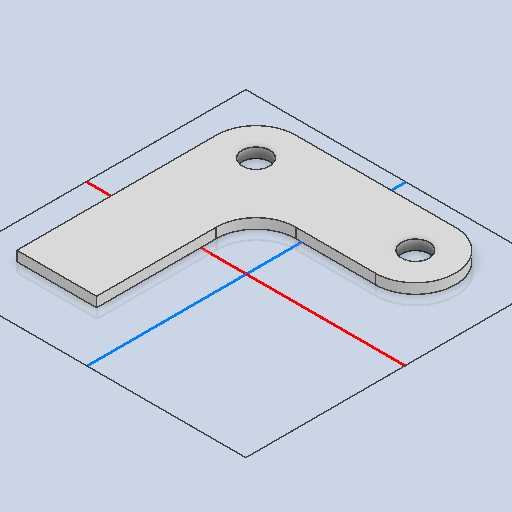
# Autodesk Inventor part: Magazine Gusset
Saved by Autodesk Inventor 2026 (Build 300175000, 175)
## iProperties
Created: 2025-04-07
Part Number: Magazine Gusset
Material: Generic
Document SubType Name: Modeling
Designer: avere
Density: 1 g/cm^3
Appearance: Default
Author: avere
Autodesk Inventor part; units mm, degrees
ref_plane "YZ Plane" through (0, 0, 0) normal (1, 0, 0) x (0, 1, 0)
ref_plane "XZ Plane" through (0, 0, 0) normal (0, 1, 0) x (-1, 0, 0)
ref_plane "XY Plane" through (0, 0, 0) normal (0, 0, 1) x (1, 0, 0)
sketch "Sketch1" plane through (0, 0, 0) normal (0, 1, 0) x (-1, 0, 0)
  circle A0 centre (13.5257, -15.1463) radius 2.1844
  circle A1 centre (-11.8743, -15.1463) radius 2.1844
  arc A2 (13.5257, -21.4963) -> (19.8757, -15.1463) centre (13.5257, -15.1463) ccw
  arc A3 (-11.8743, -8.7963) -> (-11.8743, -21.4963) centre (-11.8743, -15.1463) ccw
  line L0 (7.1757, 10.2537) -> (7.1757, -2.4463)
  line L1 (0.8257, -8.7963) -> (-11.8743, -8.7963)
  arc A4 (0.8257, -8.7963) -> (7.1757, -2.4463) centre (0.8257, -2.4463) ccw
  line L2 (19.8757, 10.2537) -> (19.8757, -15.1463)
  line L3 (13.5257, -21.4963) -> (-11.8743, -21.4963)
  line L4 (7.1757, 10.2537) -> (7.1757, 16.6037)
  line L5 (7.1757, 16.6037) -> (19.8757, 16.6037)
  line L6 (19.8757, 16.6037) -> (19.8757, 10.2537)
  point P0 (0, 0)
  dimension "d0" = 12.7
  dimension "d1" = 12.7
  dimension "d2" = 6.35
  constraints: 14 end point, 6 point on circle, 5 centre point, 4 tangent, 3 vertical, 2 coincident, 2 perpendicular
  measures "d0" diameter of A2
  measures "d1" diameter of A3
  measures "d2" radius of A4
extrude "Extrusion1" add sketch "Sketch1" along normal blind 1.5875
body "Solid1"
